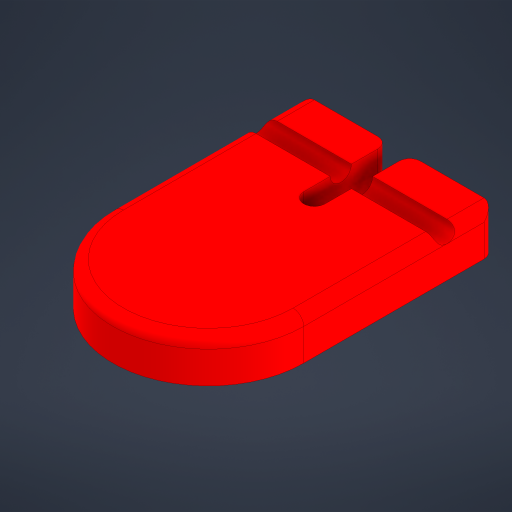
# Autodesk Inventor part: Rod_Motor_Cut_Assist_Tool
Saved by Autodesk Inventor 2023.4 (Build 274418000, 418)
## iProperties
Created: 2025-03-27
Part Number: Rod_Motor_Cut_Assist_Tool
Material: Generic
Document SubType Name: Modeling
Designer: xSibe
Density: 1 g/cm^3
Appearance: Plastic Red
Author: xSibe
Autodesk Inventor part; units mm, degrees
ref_plane "YZ Plane" through (0, 0, 0) normal (1, 0, 0) x (0, 1, 0)
ref_plane "XZ Plane" through (0, 0, 0) normal (0, 1, 0) x (-1, 0, 0)
ref_plane "XY Plane" through (0, 0, 0) normal (0, 0, 1) x (1, 0, 0)
sketch "Sketch1" plane through (0, 0, 0) normal (0, 1, 0) x (-1, 0, 0)
  line L0 (22.5, 22.5) -> (-22.5, 22.5)
  line L1 (-22.5, 22.5) -> (-22.5, -22.5)
  line L2 (-22.5, -22.5) -> (22.5, -22.5)
  line L3 (22.5, -22.5) -> (22.5, 22.5)
  line L4 (22.5, 22.5) -> (-22.5, -22.5) construction
  line L5 (-22.5, 22.5) -> (22.5, -22.5) construction
  line L6 (22.5, -22.5) -> (-22.5, -22.5)
  line L7 (-22.5, -22.5) -> (-22.5, 0)
  line L8 (-22.5, 0) -> (22.5, 0)
  line L9 (22.5, 0) -> (22.5, -22.5)
  line L10 (22.5, -11.25) -> (-22.5, -11.25)
  line L11 (22.5, -8.75) -> (-22.5, -8.75)
  line L12 (-22.5, -8.75) -> (-22.5, -13.75)
  line L13 (-22.5, -13.75) -> (22.5, -13.75)
  line L14 (22.5, -13.75) -> (22.5, -8.75)
  line L15 (22.5, -8.75) -> (-22.5, -13.75) construction
  line L16 (-22.5, -8.75) -> (22.5, -13.75) construction
  line L17 (2.5, 0) -> (-2.5, 0)
  line L18 (-2.5, 0) -> (-2.5, -22.5)
  line L19 (-2.5, -22.5) -> (2.5, -22.5)
  line L20 (2.5, -22.5) -> (2.5, 0)
  line L21 (2.5, 0) -> (-2.5, -22.5) construction
  line L22 (-2.5, 0) -> (2.5, -22.5) construction
  circle A0 centre (0, 22.5) radius 22.5
  point P0 (0, 0)
  point P1 (0, -11.25)
  point P2 (2.5, -8.75)
  point P3 (-2.5, -8.75)
  point P4 (-2.5, -13.75)
  point P5 (2.5, -13.75)
  dimension "d0" = 45
  dimension "d1" = 45
  dimension "d2" = 5
  dimension "d3" = 5
  constraints: 46 end point, 11 midpoint, 8 parallel, 4 horizontal, 4 perpendicular, 2 point on line, 3 other
  measures "d0" distance of L2.end L1.end
  measures "d1" distance of L1.end L0.end
  measures "d2" distance of L12.end L11.end
  measures "d3" distance of L19.end L18.end
extrude "Extrusion1" add sketch "Sketch1" along normal blind 7.5 contours A0 L0 | L0 A0 | L3 L8 A0 | A0 L8 L1 | L3 L11 L20 L8 | L8 L18 L11 L1 | L3 L10 L20 L11 | L11 L18 L10 L1 | L3 L13 L20 L10 | L10 L18 L13 L1 | L3 L2 L20 L13 | L13 L18 L2 L1
extrude "Extrusion2" add sketch "Sketch1" along normal blind 2.5 from surface at 7.5 contours A0 L0 | L0 A0 | L3 L8 A0 | A0 L8 L1 | L3 L11 L20 L8 | L8 L18 L11 L1 | L3 L2 L20 L13 | L13 L18 L2 L1
fillet "Fillet1" radius 2.5 15 edges at (-12.5, 7.5, -8.75) (-12.5, 7.5, -13.75) (12.5, 7.5, -13.75) (12.5, 7.5, -8.75) (0, 10, 45) (22.5, 10, 6.875) (-22.5, 10, 6.875) (-22.5, 10, -18.125) (22.5, 10, -18.125) (22.5, 5, -22.5) (-22.5, 5, -22.5) (-2.5, 5, -22.5) (2.5, 5, -22.5) (-2.5, 5, 0) (2.5, 5, 0)
body "Solid1"
